Profile Joiner - Horiz to Vert_v4 (Autodesk Fusion 360 design; units mm, degrees)
Autodesk Fusion 360 part; units mm, degrees
sketch "Sketch1" plane through (0, 0, 0) normal (0, 0, 1) x (1, 0, 0)
  line L0 (-1.8, 5.5) -> (-3.4393, 5.5)
  line L1 (-6.1, -2.8393) -> (-3.4393, -5.5)
  line L2 (-6.1, 2.8393) -> (-6.1, -2.8393)
  line L3 (-1.8, -5.5) -> (-1.8, -3.2628)
  arc A0 (-1.4586, 3.1214) -> (-1.8, 3.2628) centre (-1.6, 3.2628) cw
  arc A1 (-1.8, -3.2628) -> (-1.4586, -3.1214) centre (-1.6, -3.2628) cw
  line L4 (-3.4393, 5.5) -> (-6.1, 2.8393)
  line L5 (-3.4393, -5.5) -> (-1.8, -5.5)
  line L6 (-0.1506, 4.4312) -> (-1.4586, 3.1214)
  line L7 (-1.8, 3.2628) -> (-1.8, 5.5)
  line L8 (-1.4586, -3.1214) -> (-0.1778, -4.4022)
  line L9 (-0.0013, -4.5787) -> (-0.0013, 4.5807)
  line L10 (-0.1778, -4.4022) -> (-0.0013, -4.5787)
  line L11 (-0.1506, 4.4312) -> (-0.0013, 4.5807)
  line L12 (-6, -2.7979) -> (-3.3979, -5.4)
  line L13 (-3.3979, -5.4) -> (-1.9, -5.4)
  line L14 (-1.9, -5.4) -> (-1.9, -3.2628)
  arc A2 (-1.3879, -3.0507) -> (-1.9, -3.2628) centre (-1.6, -3.2628) ccw
  line L15 (-1.3879, -3.0507) -> (-0.1071, -4.3315)
  line L16 (-0.1071, -4.3315) -> (-0.1013, -4.3373)
  line L17 (-0.1013, -4.3373) -> (-0.1013, 4.3391)
  line L18 (-0.1013, 4.3391) -> (-1.3876, 3.0509)
  arc A3 (-1.9, 3.2628) -> (-1.3876, 3.0509) centre (-1.6, 3.2628) ccw
  line L19 (-1.9, 3.2628) -> (-1.9, 5.4)
  line L20 (-1.9, 5.4) -> (-3.3979, 5.4)
  line L21 (-3.3979, 5.4) -> (-6, 2.7979)
  line L22 (-6, 2.7979) -> (-6, -2.7979)
  line L23 (-0.1013, -4.3373) -> (-0.0013, -4.4373)
  line L24 (-0.1013, 4.3391) -> (-0.0013, 4.4391)
  dimension "d11" = -0.1
  constraint vertical L9
  constraint parallel L8 L10
  constraint parallel L6 L11
  constraint coincident L9 L23.end
  constraint parallel L15 L23
  constraint coincident L9 L24.end
  constraint perpendicular L23 L24
extrude "Extrude1" add sketch "Sketch1" along normal blind 10.8 from surface at -0.4 contours L9 L17 L23 L24 | L12 L13 L14 A2 L15 L16 L17 L18 A3 L19 L20 L21 L22
ref_plane "WorkPlane1" through (-2.649, 0, 5) normal (0, -1, 0) x (1, 0, 0)
sketch "Sketch2" plane through (-2.6197, 0, 5) normal (0, -1, 0) x (1, 0, 0)
  line L0 (4.0756, -3.1214) -> (2.7948, -4.4022)
  line L1 (4.417, -5.5) -> (4.417, -3.2628)
  line L2 (8.717, 2.8393) -> (8.717, -2.8393)
  line L3 (6.0564, 5.5) -> (8.717, 2.8393)
  line L4 (2.7677, 4.4312) -> (2.6183, 4.5807)
  line L5 (2.6183, -4.5787) -> (2.6183, 4.5807)
  line L6 (2.7677, 4.4312) -> (4.0756, 3.1214)
  line L7 (4.417, 3.2628) -> (4.417, 5.5)
  arc A0 (4.0756, 3.1214) -> (4.417, 3.2628) centre (4.217, 3.2628) ccw
  line L8 (2.7948, -4.4022) -> (2.6183, -4.5787)
  line L9 (6.0564, -5.5) -> (4.417, -5.5)
  line L10 (4.417, 5.5) -> (6.0564, 5.5)
  line L11 (8.717, -2.8393) -> (6.0564, -5.5)
  line L12 (4.0756, -3.1214) -> (4.417, -2.78)
  line L13 (4.417, -3.2628) -> (4.417, -2.78)
  line L14 (2.7183, -4.3373) -> (2.7183, 4.3391)
  line L15 (2.7241, -4.3315) -> (2.7183, -4.3373)
  line L16 (4.0049, -3.0507) -> (2.7241, -4.3315)
  line L17 (4.0049, -3.0507) -> (4.517, -2.5386)
  line L18 (4.517, -3.2628) -> (4.517, -2.5386)
  line L19 (4.517, -5.4) -> (4.517, -3.2628)
  line L20 (6.0149, -5.4) -> (4.517, -5.4)
  line L21 (8.617, -2.7979) -> (6.0149, -5.4)
  line L22 (8.617, 2.7979) -> (8.617, -2.7979)
  line L23 (6.0149, 5.4) -> (8.617, 2.7979)
  line L24 (4.517, 5.4) -> (6.0149, 5.4)
  line L25 (4.517, 3.2628) -> (4.517, 5.4)
  arc A1 (4.0048, 3.0508) -> (4.517, 3.2628) centre (4.217, 3.2628) ccw
  line L26 (2.7183, 4.3391) -> (4.0048, 3.0508)
  line L27 (2.7241, -4.3315) -> (2.5161, -4.5395)
  line L28 (2.5161, -4.5395) -> (2.5161, 4.6831)
  line L29 (2.5161, 4.6831) -> (2.6183, 4.5807)
  line L30 (2.7183, 4.3391) -> (2.6183, 4.4392)
  point P0 (2.617, 0)
  dimension "d12" = 0.1
  constraint parallel L0 L8
  constraint parallel L4 L6
  constraint parallel L0 L12
  constraint parallel L1 L13
  constraint parallel L16 L27
  constraint parallel L5 L28
  constraint parallel L4 L29
  constraint coincident L5 L30.end
  constraint parallel L26 L30
extrude "Extrude2" add sketch "Sketch2" along normal mid plane 8.8744 contours L5 L14 L27 L30 | L14 L15 L16 L17 L18 L19 L20 L21 L22 L23 L24 L25 A1 L26 L27
